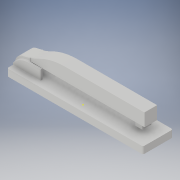
# Autodesk Inventor part: Stapler
Saved by Autodesk Inventor 2017 (Build 210142000, 142)
## iProperties
Created: 2018-03-21
Part Number: Stapler
Material: Generic
Document SubType Name: Modeling
Designer: landontracy
Density: 1 g/cm^3
Appearance: Default
Author: landontracy
Autodesk Inventor part; units mm, degrees
ref_plane "YZ Plane" through (0, 0, 0) normal (1, 0, 0) x (0, 1, 0)
ref_plane "XZ Plane" through (0, 0, 0) normal (0, 1, 0) x (-1, 0, 0)
ref_plane "XY Plane" through (0, 0, 0) normal (0, 0, 1) x (1, 0, 0)
sketch "Stapler Bottom" plane through (0, 0, 0) normal (0, 1, 0) x (-1, 0, 0)
  line L0 (94.8504, -32.7544) -> (-89.2889, -32.7544)
  line L1 (-90.2889, -31.6958) -> (-90.2889, 7.1831)
  line L2 (-89.8327, 8.1831) -> (94.7084, 8.1831)
  line L3 (95.8504, 7.1831) -> (95.8504, -30.3771)
  line L4 (95.8504, 7.1831) -> (94.7084, 8.1831)
  line L5 (95.8504, -30.3771) -> (94.8504, -32.7544)
  line L6 (-89.2889, -32.7544) -> (-90.2889, -31.6958)
  line L7 (-90.2889, 7.1831) -> (-89.8327, 8.1831)
  point P0 (0, 0)
  dimension "d2" = 1
  dimension "d3" = 1
  dimension "d4" = 1
  dimension "d5" = 1
  dimension "d6" = 38.8788
  dimension "d7" = 184.5411
  constraints: 16 end point, 2 parallel, 1 horizontal, 1 perpendicular
  measures "d2" vertical distance of L3.start L2.end
  measures "d3" horizontal distance of L3.end L0.start
  measures "d4" horizontal distance of L0.end L1.start
  measures "d5" vertical distance of L1.end L2.start
  measures "d6" distance of L1.start L1.end
  measures "d7" distance of L2.start L2.end
extrude "Extrusion1" add sketch "Stapler Bottom" along normal blind 9.52
fillet "Fillet1" radius 2 8 edges at (89.8327, 4.76, 8.1831) (90.2889, 4.76, 7.1831) (89.2889, 4.76, -32.7544) (90.2889, 4.76, -31.6958) (-94.8504, 4.76, -32.7544) (-95.8504, 4.76, -30.3771) (-95.8504, 4.76, 7.1831) (-94.7084, 4.76, 8.1831)
sketch "Sketch3" plane through (0, 9.52, 0) normal (0, 1, 0) x (1, 0, 0)
  point P0 (0, 0)
sketch "Sketch4" plane through (0, 9.52, 0) normal (0, 1, 0) x (1, 0, 0)
  line L0 (-95.8504, 29.9736) -> (-95.8504, -6.1831) projected
  line L1 (-95.8504, 0) -> (-73.8768, 0)
  line L2 (-73.8768, 2.5226) -> (-95.8504, 2.5226)
  line L3 (-95.8504, 2.5226) -> (-95.8504, 0)
  line L4 (-95.8504, 11.8953) -> (-84.8636, 11.8953)
  line L5 (-95.8504, 23.7905) -> (-73.8768, 23.7905)
  line L6 (-73.8768, 21.2679) -> (-95.8504, 21.2679)
  line L7 (-95.8504, 21.2679) -> (-95.8504, 23.7905)
  line L8 (-73.8768, 23.7905) -> (-57.9869, 23.7905)
  line L9 (-73.8768, 21.2679) -> (-57.9869, 21.2679)
  line L10 (-57.9869, 21.2679) -> (-57.9869, 23.7905)
  line L11 (-73.8768, 2.5226) -> (-57.9869, 2.5226)
  line L12 (-73.8768, 0) -> (-57.9869, 0)
  line L13 (-57.9869, 0) -> (-57.9869, 2.5226)
  point P0 (0, 0)
  constraints: 26 end point, 6 horizontal, 4 symmetric about line, 3 perpendicular, 1 midpoint, 1 parallel, 1 point on line
extrude "Extrusion2" add sketch "Sketch4" along normal blind 13.175
sketch "Sketch5" plane through (-95.8504, 9.52, 0) normal (0, 0, 1) x (1, 0, 0)
  line L0 (0, 0) -> (0, 13.175) projected
  line L1 (0, 2.7215) -> (7.1075, 13.175)
  line L2 (0, 13.175) -> (37.8635, 13.175) projected
  line L3 (7.1075, 13.175) -> (0, 13.175)
  line L4 (0, 13.175) -> (0, 2.7215)
  point P0 (95.8504, -9.52)
  constraints: 6 end point, 2 point on line, 1 horizontal, 1 perpendicular
extrude "Extrusion3" cut sketch "Sketch5" against normal blind 32.225
fillet "Fillet2" radius 25.8125 2 edges at (-88.7429, 22.695, -1.2613) (-88.7429, 22.695, -22.5292)
sketch "Sketch6" plane through (0, 9.52, 0) normal (0, 1, 0) x (1, 0, 0)
  line L0 (-75.1046, 0) -> (-75.1046, 2.5226) projected
  line L1 (-95.5889, 21.3653) -> (-75.1046, 21.3653)
  line L2 (-75.1046, 21.3653) -> (-75.1046, 2.5226)
  line L3 (-75.1046, 2.5226) -> (-95.5889, 2.5226)
  line L4 (-95.5889, 2.5226) -> (-95.5889, 21.3653)
  point P0 (0, 0)
  constraints: 8 end point, 2 parallel, 1 horizontal, 1 perpendicular
extrude "Extrusion4" add sketch "Sketch6" along normal blind 14.7625
fillet "Fillet3" radius 13.1125 1 edges at (-95.5889, 24.2825, -11.944)
sketch "Sketch7" plane through (-75.1046, 9.52, -2.5226) normal (1, 0, 0) x (0, 0, -1)
  line L0 (0.7655, 13.9146) -> (18.1457, 13.9146)
  line L1 (18.1457, 13.9146) -> (18.1457, 5.7203)
  line L2 (0.7655, 5.7203) -> (0.7655, 13.9146)
  line L3 (0.7655, 10.1654) -> (18.1457, 10.1654)
  point P0 (-2.5226, -9.52)
  constraints: 8 end point, 2 perpendicular, 2 point on line, 1 horizontal, 1 parallel
extrude "Extrusion5" add sketch "Sketch7" along normal blind 156.05
sketch "Sketch8" plane through (-75.1046, 23.4346, -3.2882) normal (0, 1, 0) x (1, 0, 0)
  line L0 (0, 17.3802) -> (156.05, 17.3802) projected
  line L1 (0, 0) -> (156.05, 0) projected
  line L2 (156.05, 17.3802) -> (0, 17.3802)
  line L3 (0, 17.3802) -> (0, 0)
  line L4 (0, 0) -> (156.05, 0)
  line L5 (156.05, 0) -> (156.05, 17.3802)
  point P0 (75.1046, -3.2882)
  constraints: 8 end point, 2 parallel, 1 horizontal, 1 perpendicular
extrude "Extrusion6" add sketch "Sketch8" along normal blind 16.35
fillet "Fillet4" radius 78.2 1 edges at (-75.1046, 39.7846, -11.9783)
fillet "Fillet5" radius 78.2 1 edges at (-75.1046, 24.2825, -11.9783)
fillet "Fillet6" radius 0.4125 9 edges at (-46.6521, 37.6173, -3.2882) (-69.4229, 28.6912, -3.2882) (26.2882, 39.7846, -3.2882) (80.9454, 39.7846, -11.9783) (-46.6521, 37.6173, -20.6684) (-69.4229, 28.6912, -20.6684) (26.2882, 39.7846, -20.6684) (80.9454, 29.735, -3.2882) (80.9454, 29.735, -20.6684)
fillet "Fillet7" radius 0.4125 7 edges at (-66.5457, 22.695, -21.2679) (-86.72, 19.9339, -23.7905) (-66.5457, 22.695, -23.7905) (-86.72, 19.9339, 0) (-66.5457, 22.695, 0) (-66.5457, 22.695, -2.5226) (-86.4593, 20.0635, -2.5226)
fillet "Fillet8" radius 0.4125 1 edges at (-95.8504, 9.52, -11.8953)
fillet "Fillet9" radius 146.4625 1 edges at (-95.5889, 9.52, -11.8953)
sketch "Sketch9" plane through (80.9454, 9.52, -2.5226) normal (1, 0, 0) x (0, 0, -1)
  line L0 (0.7655, 10.1654) -> (0.7655, 16.6266) projected
  line L1 (18.1457, 10.1654) -> (0.7655, 10.1654) projected
  line L2 (18.1457, 12.5223) -> (18.1457, 10.1654)
  line L3 (18.1457, 10.1654) -> (0.7655, 10.1654)
  line L4 (0.7655, 10.1654) -> (0.7655, 12.5223)
  line L5 (0.7655, 12.5223) -> (18.1457, 12.5223)
  line L6 (18.1457, 16.6266) -> (18.1457, 10.1654) projected
  point P0 (-2.5226, -9.52)
  constraints: 8 end point, 1 parallel, 1 perpendicular, 1 point on line
extrude "Extrusion7" cut sketch "Sketch9" against normal blind 156.05
sketch "Sketch10" plane through (80.9454, 22.0423, -20.2559) normal (0, -1, 0) x (1, 0, 0)
  line L0 (-5.4077, 14.5777) -> (-14.9652, 14.5777)
  line L1 (-14.9652, 14.5777) -> (-14.9652, 2.2698)
  line L2 (-14.9652, 2.2698) -> (-5.4077, 2.2698)
  line L3 (-5.4077, 2.2698) -> (-5.4077, 14.5777)
  point P0 (-80.9454, 20.2559)
  constraints: 8 end point, 2 parallel, 1 horizontal, 1 perpendicular
extrude "Extrusion8" add sketch "Sketch10" along normal blind 6.825
sketch "Sketch11" plane through (75.5377, 22.0423, -5.6781) normal (1, 0, 0) x (0, 0, -1)
  line L0 (-2.39, 0) -> (14.9902, 0) projected
  line L1 (0, -6.825) -> (12.3079, -6.825) projected
  circle A0 centre (3.0482, -3.3444) radius 1.2025
  circle A1 centre (9.4058, -3.4806) radius 1.2025
  point P0 (-5.6781, -22.0423)
  constraints: 2 centre point
extrude "Extrusion9" cut sketch "Sketch11" against normal blind 2.0625
body "Solid1"
